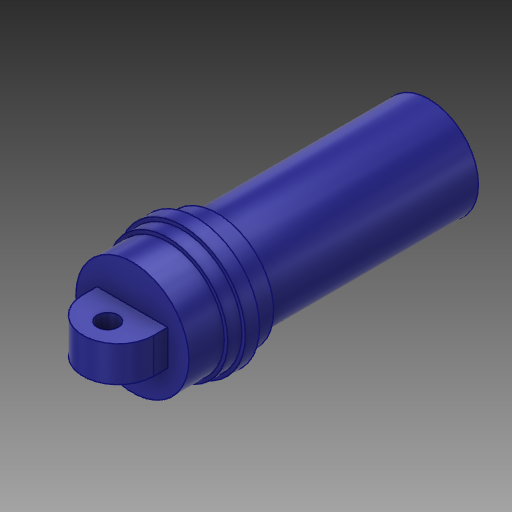
# Autodesk Inventor part: タミヤダンパー
Saved by Autodesk Inventor 2017 (Build 210142000, 142)
## iProperties
Part Number: タミヤダンパー
Material: 一般
Document SubType Name: Modeling
Designer: 雪村
Density: 1 g/cm^3
Appearance: 滑らか - 濃紺色
Mass: 6.86149 g
Surface Area: 31.2175 cm^2
Volume: 6.86149 cm^3
Author: 雪村
Autodesk Inventor part; units mm, degrees
ref_plane "YZ Plane" through (0, 0, 0) normal (1, 0, 0) x (0, 1, 0)
ref_plane "XZ Plane" through (0, 0, 0) normal (0, 1, 0) x (-1, 0, 0)
ref_plane "XY Plane" through (0, 0, 0) normal (0, 0, 1) x (1, 0, 0)
sketch "スケッチ1" plane through (0, 0, 0) normal (0, 0, 1) x (1, 0, 0)
  circle A0 centre (0, 0) radius 7
  circle A1 centre (0, 0) radius 2.5
  dimension "d0" = 14
  dimension "d1" = 5
  constraints: 2 centre point, 2 coincident
  measures "d0" diameter of A0
  measures "d1" diameter of A1
extrude "押し出し1" add sketch "スケッチ1" along normal blind 30
sketch "スケッチ2" plane through (0, 0, 30) normal (0, 0, 1) x (1, 0, 0)
  circle A0 centre (0, 0) radius 8
  dimension "d4" = 16
  constraints: 1 centre point, 1 coincident
  measures "d4" diameter of A0
extrude "押し出し2" add sketch "スケッチ2" along normal blind 3
sketch "スケッチ3" plane through (0, 0, 33) normal (0, 0, 1) x (1, 0, 0)
  circle A0 centre (0, 0) radius 9
  dimension "d7" = 18
  constraints: 1 centre point, 1 coincident
  measures "d7" diameter of A0
extrude "押し出し3" add sketch "スケッチ3" along normal blind 2
sketch "スケッチ4" plane through (0, 0, 35) normal (0, 0, 1) x (1, 0, 0)
  circle A0 centre (0, 0) radius 8.5
  dimension "d10" = 17
  constraints: 1 centre point, 1 coincident
  measures "d10" diameter of A0
extrude "押し出し4" add sketch "スケッチ4" along normal blind 2
sketch "スケッチ5" plane through (0, 0, 37) normal (0, 0, 1) x (1, 0, 0)
  circle A0 centre (0, 0) radius 8
  dimension "d13" = 16
  constraints: 1 centre point, 1 coincident
  measures "d13" diameter of A0
extrude "押し出し5" add sketch "スケッチ5" along normal blind 5
sketch "スケッチ6" plane through (0, 0, 42) normal (0, 0, 1) x (1, 0, 0)
  line L0 (-5, -2.5) -> (5, -2.5)
  line L1 (5, -2.5) -> (5, 2.5)
  line L2 (5, 2.5) -> (-5, 2.5)
  line L3 (-5, 2.5) -> (-5, -2.5)
  line L4 (-5, -2.5) -> (5, 2.5) construction
  line L5 (5, -2.5) -> (-5, 2.5) construction
  point P0 (0, 0)
  dimension "d16" = 10
  dimension "d17" = 5
  constraints: 12 end point, 2 horizontal, 2 midpoint, 2 vertical
  measures "d16" distance of L2.end L1.end
  measures "d17" distance of L1.end L0.end
extrude "押し出し6" add sketch "スケッチ6" along normal blind 7
fillet "フィレット1" radius 5 1 edges at (-5, 0, 49)
fillet "フィレット2" radius 5 1 edges at (5, 0, 49)
sketch "スケッチ7" plane through (-5, -2.5, 42) normal (0, -1, 0) x (1, 0, 0)
  arc A0 (10, 2) -> (0, 2) centre (5, 2) ccw projected
  line L0 (0, 0) -> (0, 2) projected
  line L1 (10, 0) -> (0, 0) projected
  line L2 (10, 0) -> (10, 2) projected
  circle A1 centre (5, 3.5) radius 1.5
  point P0 (5, -42)
  dimension "d22" = 3
  dimension "d23" = 2
  constraints: 1 centre point, 1 vertical alignment
  measures "d22" diameter of A1
extrude "押し出し7" cut sketch "スケッチ7" against normal blind 8 contours A1
